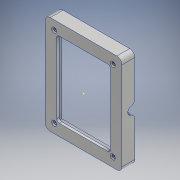
# Autodesk Inventor part: cardboardmountfront_sjc
Saved by Autodesk Inventor 2017 SP1 (Build 210196100, 196)
## iProperties
Created: 2017-04-07
Part Number: cardboardmountfront_sjc
Material: Generic
Document SubType Name: Modeling
Designer: Sam
Density: 1 g/cm^3
Appearance: Aluminum - Flat
Author: Sam
Autodesk Inventor part; units mm, degrees
ref_plane "YZ Plane" through (0, 0, 0) normal (1, 0, 0) x (0, 1, 0)
ref_plane "XZ Plane" through (0, 0, 0) normal (0, 1, 0) x (-1, 0, 0)
ref_plane "XY Plane" through (0, 0, 0) normal (0, 0, 1) x (1, 0, 0)
sketch "Sketch1" plane through (0, 0, 0) normal (0, 1, 0) x (-1, 0, 0)
  line L0 (-30, 38.5) -> (30, 38.5)
  line L1 (30, 38.5) -> (30, -38.5)
  line L2 (30, -38.5) -> (-30, -38.5)
  line L3 (-30, -38.5) -> (-30, 38.5)
  line L4 (-30, 38.5) -> (30, -38.5) construction
  line L5 (30, 38.5) -> (-30, -38.5) construction
  point P0 (0, 0)
  dimension "d0" = 60
  dimension "d1" = 77
  constraints: 12 end point, 2 midpoint, 2 parallel, 1 horizontal, 1 perpendicular
  measures "d0" distance of L1.end L2.end
  measures "d1" distance of L0.end L1.end
extrude "Extrusion1" add sketch "Sketch1" along normal blind 10
sketch "Sketch2" plane through (0, 10, 0) normal (0, 1, 0) x (1, 0, 0)
  line L0 (27, -35.5) -> (-27, -35.5)
  line L1 (-27, -35.5) -> (-27, 35.5)
  line L2 (-27, 35.5) -> (27, 35.5)
  line L3 (27, 35.5) -> (27, -35.5)
  line L4 (27, -35.5) -> (-27, 35.5) construction
  line L5 (-27, -35.5) -> (27, 35.5) construction
  point P0 (0, 0)
  dimension "d4" = 54
  dimension "d5" = 71
  constraints: 12 end point, 2 midpoint, 2 parallel, 1 horizontal, 1 perpendicular
  measures "d4" distance of L1.end L2.end
  measures "d5" distance of L0.end L1.end
extrude "Extrusion2" cut sketch "Sketch2" against normal blind 8
sketch "Sketch3" plane through (0, 2, 0) normal (0, 1, 0) x (1, 0, 0)
  line L0 (21, -29.5) -> (-21, -29.5)
  line L1 (-21, -29.5) -> (-21, 29.5)
  line L2 (-21, 29.5) -> (21, 29.5)
  line L3 (21, 29.5) -> (21, -29.5)
  line L4 (21, -29.5) -> (-21, 29.5) construction
  line L5 (-21, -29.5) -> (21, 29.5) construction
  point P0 (0, 0)
  dimension "d8" = 42
  dimension "d9" = 59
  constraints: 12 end point, 2 midpoint, 2 parallel, 1 horizontal, 1 perpendicular
  measures "d8" distance of L1.end L2.end
  measures "d9" distance of L0.end L1.end
extrude "Extrusion3" cut sketch "Sketch3" against normal blind 7
fillet "Fillet1" radius 4 4 edges at (-30, 5, 38.5) (30, 5, 38.5) (-30, 5, -38.5) (30, 5, -38.5)
sketch "Sketch4" plane through (0, 0, 0) normal (0, -1, 0) x (1, 0, 0)
  point P0 (0, 0)
sketch "Sketch5" plane through (0, 0, 0) normal (0, -1, 0) x (1, 0, 0)
  point P0 (0, 0)
  point P1 (22.809, 31.309)
  point P2 (22.809, -31.309)
  point P3 (-23, 31.5)
  point P4 (-23, -31.5)
hole "Hole1" at (22.809, 0, 31.309) at (22.809, 0, -31.309) at (-23, 0, -31.5) at (-23, 0, 31.5) direction (0, 1, 0) diameter 2.459 depth 8.8 tip angle 118 countersink diameter 4 countersink angle 90 thread size "M3x0.5" class "6H" standard "ANSI Metric M Profile"
sketch "Sketch7" plane through (30, 0, 34.5) normal (1, 0, 0) x (0, 0, -1)
  point P0 (34.5, 0)
  point P1 (34.5, 7.5)
hole "Hole2" at (30, 7.5, 0) direction (-1, 0, 0) diameter 6 depth 8.8 tip angle 118
fillet "Fillet2" radius 4 2 edges at (28.5, 10, -1.6583) (28.5, 10, 1.6583)
fillet "Fillet3" radius 2 1 edges at (-21, 1, -29.5)
fillet "Fillet4" radius 2 1 edges at (-21, 1, 29.5)
fillet "Fillet5" radius 2 1 edges at (21, 1, 29.5)
fillet "Fillet6" radius 2 1 edges at (21, 1, -29.5)
equation "\"x\" = 54"
equation "\"z\" = 71"
equation "\"hole\" = 4"
body "Solid1"
